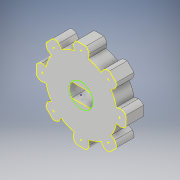
# Autodesk Inventor part: 8 ul Driver Gear
Saved by Autodesk Inventor 2017 (Build 210142000, 142)
## iProperties
Created: 2018-03-04
Part Number: 8 ul Driver Gear
Material: Generic
Document SubType Name: Modeling
Designer: Russ
Density: 1 g/cm^3
Appearance: Default
Author: Russ
Autodesk Inventor part; units mm, degrees
ref_plane "YZ Plane" through (0, 0, 0) normal (1, 0, 0) x (0, 1, 0)
ref_plane "XZ Plane" through (0, 0, 0) normal (0, 1, 0) x (-1, 0, 0)
ref_plane "XY Plane" through (0, 0, 0) normal (0, 0, 1) x (1, 0, 0)
sketch "Sketch1" plane through (0, 0, 0) normal (0, 0, 1) x (1, 0, 0)
  arc A0 (-2.0086, 7.3505) -> (2.0086, 7.3505) centre (0, 0) ccw
  line L0 (0, 7.62) -> (0, 9.525)
  line L1 (0, 9.525) -> (1.016, 9.525)
  line L2 (0, 9.525) -> (-1.016, 9.525)
  arc A1 (-1.4866, 7.4736) -> (1.4866, 7.4736) centre (0, 0) ccw
  line L3 (-1.4866, 7.4736) -> (-1.8582, 9.342)
  line L4 (-2.916, 7.04) -> (-3.6451, 8.8)
  line L5 (-4.2334, 6.3358) -> (-5.2918, 7.9197)
  line L6 (-5.3882, 5.3882) -> (-6.7352, 6.7352)
  line L7 (-6.3358, 4.2334) -> (-7.9197, 5.2918)
  line L8 (-7.04, 2.916) -> (-8.8, 3.6451)
  line L9 (-7.04, -2.916) -> (-8.8, -3.6451)
  line L10 (-6.3358, -4.2334) -> (-7.9197, -5.2918)
  line L11 (-5.3882, -5.3882) -> (-6.7352, -6.7352)
  line L12 (-4.2334, -6.3358) -> (-5.2918, -7.9197)
  line L13 (-2.916, -7.04) -> (-3.6451, -8.8)
  line L14 (-1.4866, -7.4736) -> (-1.8582, -9.342)
  line L15 (0, -7.62) -> (0, -9.525)
  line L16 (1.4866, -7.4736) -> (1.8582, -9.342)
  line L17 (2.916, -7.04) -> (3.6451, -8.8)
  line L18 (4.2334, -6.3358) -> (5.2918, -7.9197)
  line L19 (5.3882, -5.3882) -> (6.7352, -6.7352)
  line L20 (6.3358, -4.2334) -> (7.9197, -5.2918)
  line L21 (7.04, -2.916) -> (8.8, -3.6451)
  line L22 (7.4736, -1.4866) -> (9.342, -1.8582)
  line L23 (7.62, 0) -> (9.525, 0)
  line L24 (7.4736, 1.4866) -> (9.342, 1.8582)
  line L25 (7.04, 2.916) -> (8.8, 3.6451)
  line L26 (6.3358, 4.2334) -> (7.9197, 5.2918)
  line L27 (5.3882, 5.3882) -> (6.7352, 6.7352)
  line L28 (4.2334, 6.3358) -> (5.2918, 7.9197)
  line L29 (2.916, 7.04) -> (3.6451, 8.8)
  line L30 (1.4866, 7.4736) -> (1.8582, 9.342)
  arc A2 (-1.4866, 7.4736) -> (1.4866, 7.4736) centre (0, 0) ccw
  arc A3 (-1.016, 9.525) -> (-1.6724, 8.4079) centre (-0.1056, 8.2386) ccw
  arc A4 (1.6724, 8.4079) -> (1.016, 9.525) centre (0.1056, 8.2386) ccw
  circle A5 centre (0, 0) radius 7.62
  line L31 (-1.4866, 7.4736) -> (-1.6724, 8.4079)
  line L32 (-1.016, 9.525) -> (1.016, 9.525)
  line L33 (1.6724, 8.4079) -> (1.4866, 7.4736)
  arc A6 (-1.016, 9.525) -> (-1.6724, 8.4079) centre (-0.1056, 8.2386) ccw
  arc A7 (1.6724, 8.4079) -> (1.016, 9.525) centre (0.1056, 8.2386) ccw
  point P0 (-7.4736, 1.4866)
  point P1 (-7.62, 0)
  point P2 (-7.4736, -1.4866)
  dimension "d0" = 15.24
  dimension "d1" = 360
  dimension "d2" = 1.016
  dimension "d3" = 1.016
  dimension "d4" = 1.905
  constraints: 68 end point, 14 point on circle, 7 centre point, 5 symmetric about line, 4 coincident, 3 concentric, 2 collinear, 1 perpendicular, 1 point on line, 1 vertical, 4 other
  measures "d0" diameter of A0
  measures "d2" distance of L1.start L1.end
  measures "d3" distance of L1.start L2.end
  measures "d4" distance of L0.start L1.start
extrude "Extrusion1" add sketch "Sketch1" along normal blind 3.81
pattern_circular "Circular Pattern1" count 8 over 360 about axis through (0, 0, 0) along (0, 0, 1) of "Extrusion1"
sketch "Sketch3" plane through (0, 0, 3.81) normal (0, 0, 1) x (1, 0, 0)
  line L0 (0, 0) -> (0, 1.5)
  line L1 (0, 1.5) -> (2, 1.5)
  line L2 (0, 1.5) -> (-2, 1.5)
  line L3 (0, 0) -> (0.1755, 0)
  line L4 (0, -1.5) -> (2, -1.5)
  line L5 (0, -1.5) -> (-2, -1.5)
  arc A0 (-2, 1.5) -> (-2, -1.5) centre (0, 0) ccw
  arc A1 (2, -1.5) -> (2, 1.5) centre (0, 0) ccw
  dimension "d14" = 1.5
  constraints: 12 end point, 4 point on circle, 4 symmetric about line, 2 centre point, 1 coincident, 1 horizontal, 1 perpendicular, 1 vertical
  measures "d14" distance from line of point (0, 0) L1
extrude "Extrusion3" cut sketch "Sketch3" against normal up to next
sketch "Sketch4" plane through (0, 0, 3.81) normal (0, 0, 1) x (1, 0, 0)
  circle A0 centre (0, 0) radius 2.5
  constraints: 1 centre point, 1 coincident
sketch "Sketch5" plane through (0, 0, 3.81) normal (0, 0, 1) x (1, 0, 0)
  arc A0 (-2, 1.5) -> (-2, -1.5) centre (0, 0) ccw projected
  line L0 (-2, 1.5) -> (2, 1.5) projected
  arc A1 (2, -1.5) -> (2, 1.5) centre (0, 0) ccw projected
  line L1 (2, -1.5) -> (-2, -1.5) projected
  line L2 (1.4866, 7.4736) -> (1.6724, 8.4079) projected
  arc A2 (1.6724, 8.4079) -> (1.016, 9.525) centre (0.1056, 8.2386) ccw projected
  line L3 (1.016, 9.525) -> (-1.016, 9.525) projected
  arc A3 (-1.016, 9.525) -> (-1.6724, 8.4079) centre (-0.1056, 8.2386) ccw projected
  line L4 (-1.6724, 8.4079) -> (-1.4866, 7.4736) projected
  arc A4 (-1.4866, 7.4736) -> (-4.2334, 6.3358) centre (0, 0) ccw projected
  line L5 (-4.2334, 6.3358) -> (-4.7627, 7.1279) projected
  arc A5 (-4.7627, 7.1279) -> (-6.0168, 7.4536) centre (-5.7509, 5.9002) ccw projected
  line L6 (-6.0168, 7.4536) -> (-7.4536, 6.0168) projected
  arc A6 (-7.4536, 6.0168) -> (-7.1279, 4.7627) centre (-5.9002, 5.7509) ccw projected
  line L7 (-7.1279, 4.7627) -> (-6.3358, 4.2334) projected
  arc A7 (-6.3358, 4.2334) -> (-7.4736, 1.4866) centre (0, 0) ccw projected
  line L8 (-7.4736, 1.4866) -> (-8.4079, 1.6724) projected
  arc A8 (-8.4079, 1.6724) -> (-9.525, 1.016) centre (-8.2386, 0.1056) ccw projected
  line L9 (-9.525, 1.016) -> (-9.525, -1.016) projected
  arc A9 (-9.525, -1.016) -> (-8.4079, -1.6724) centre (-8.2386, -0.1056) ccw projected
  line L10 (-8.4079, -1.6724) -> (-7.4736, -1.4866) projected
  arc A10 (-7.4736, -1.4866) -> (-6.3358, -4.2334) centre (0, 0) ccw projected
  line L11 (-6.3358, -4.2334) -> (-7.1279, -4.7627) projected
  arc A11 (-7.1279, -4.7627) -> (-7.4536, -6.0168) centre (-5.9002, -5.7509) ccw projected
  line L12 (-7.4536, -6.0168) -> (-6.0168, -7.4536) projected
  arc A12 (-6.0168, -7.4536) -> (-4.7627, -7.1279) centre (-5.7509, -5.9002) ccw projected
  line L13 (-4.7627, -7.1279) -> (-4.2334, -6.3358) projected
  arc A13 (-4.2334, -6.3358) -> (-1.4866, -7.4736) centre (0, 0) ccw projected
  line L14 (-1.4866, -7.4736) -> (-1.6724, -8.4079) projected
  arc A14 (-1.6724, -8.4079) -> (-1.016, -9.525) centre (-0.1056, -8.2386) ccw projected
  line L15 (-1.016, -9.525) -> (1.016, -9.525) projected
  arc A15 (1.016, -9.525) -> (1.6724, -8.4079) centre (0.1056, -8.2386) ccw projected
  line L16 (1.6724, -8.4079) -> (1.4866, -7.4736) projected
  arc A16 (1.4866, -7.4736) -> (4.2334, -6.3358) centre (0, 0) ccw projected
  line L17 (4.2334, -6.3358) -> (4.7627, -7.1279) projected
  arc A17 (4.7627, -7.1279) -> (6.0168, -7.4536) centre (5.7509, -5.9002) ccw projected
  line L18 (6.0168, -7.4536) -> (7.4536, -6.0168) projected
  arc A18 (7.4536, -6.0168) -> (7.1279, -4.7627) centre (5.9002, -5.7509) ccw projected
  line L19 (7.1279, -4.7627) -> (6.3358, -4.2334) projected
  arc A19 (6.3358, -4.2334) -> (7.4736, -1.4866) centre (0, 0) ccw projected
  line L20 (7.4736, -1.4866) -> (8.4079, -1.6724) projected
  arc A20 (8.4079, -1.6724) -> (9.525, -1.016) centre (8.2386, -0.1056) ccw projected
  line L21 (9.525, -1.016) -> (9.525, 1.016) projected
  arc A21 (9.525, 1.016) -> (8.4079, 1.6724) centre (8.2386, 0.1056) ccw projected
  line L22 (8.4079, 1.6724) -> (7.4736, 1.4866) projected
  arc A22 (7.4736, 1.4866) -> (6.3358, 4.2334) centre (0, 0) ccw projected
  line L23 (6.3358, 4.2334) -> (7.1279, 4.7627) projected
  arc A23 (7.1279, 4.7627) -> (7.4536, 6.0168) centre (5.9002, 5.7509) ccw projected
  line L24 (7.4536, 6.0168) -> (6.0168, 7.4536) projected
  arc A24 (6.0168, 7.4536) -> (4.7627, 7.1279) centre (5.7509, 5.9002) ccw projected
  line L25 (4.7627, 7.1279) -> (4.2334, 6.3358) projected
  arc A25 (4.2334, 6.3358) -> (1.4866, 7.4736) centre (0, 0) ccw projected
body "Solid1"
